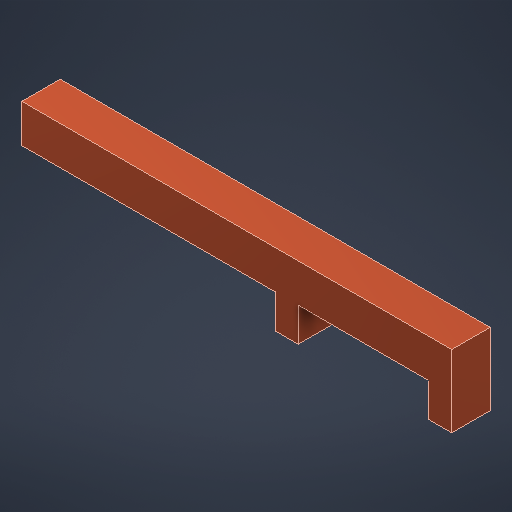
# Autodesk Inventor part: Bus_copper_GND
Saved by Autodesk Inventor 2026.2 (Build 302298000, 298)
## iProperties
Created: 2025-12-09
Part Number: Bus_copper_GND
Material: Медь
Document SubType Name: Modeling
Designer: EV-TECH
Density: 8.94 g/cm^3
Appearance: Медь — сатинированная
Author: EV-TECH
Autodesk Inventor part; units mm, degrees
ref_plane "YZ Plane" through (0, 0, 0) normal (1, 0, 0) x (0, 1, 0)
ref_plane "XZ Plane" through (0, 0, 0) normal (0, 1, 0) x (-1, 0, 0)
ref_plane "XY Plane" through (0, 0, 0) normal (0, 0, 1) x (1, 0, 0)
sketch "Эскиз1" plane through (0, 0, 0) normal (0, 1, 0) x (-1, 0, 0)
  line L0 (0, 0) -> (3, 0)
  line L1 (3, 0) -> (3, -5)
  line L2 (3, -5) -> (0, -5)
  line L3 (0, -5) -> (0, 0)
  line L4 (3, 0) -> (23, 0)
  line L5 (23, 0) -> (20, 0)
  line L6 (20, 0) -> (20, -5)
  line L7 (20, -5) -> (23, -5)
  line L8 (23, -5) -> (23, 0)
  point P0 (17, 0)
  dimension "d0" = 3
  dimension "d1" = 5
  dimension "d17" = 20
  dimension "d18" = 3
  dimension "d19" = 5
  constraints: 18 end point, 4 parallel, 3 horizontal, 2 perpendicular, 1 point on line
  measures "d0" distance of L1.end L2.end
  measures "d1" distance of L0.end L1.end
  measures "d17" distance of L0.end L4.end
  measures "d18" distance of L6.end L7.end
  measures "d19" distance of L7.end L4.end
extrude "Выдавливание1" add sketch "Эскиз1" along normal blind 4.4
sketch "Эскиз2" plane through (0, 4.4, 0) normal (0, 1, 0) x (1, 0, 0)
  line L0 (0, 0) -> (-56, 0)
  line L1 (-56, 0) -> (-56, 5)
  line L2 (-56, 5) -> (0, 5)
  line L3 (0, 5) -> (0, 0)
  dimension "d13" = 5
  dimension "d14" = 56
  constraints: 8 end point, 2 parallel, 1 horizontal, 1 perpendicular
  measures "d13" distance of L0.end L1.end
  measures "d14" distance of L1.end L2.end
extrude "Выдавливание2" add sketch "Эскиз2" along normal blind 5
